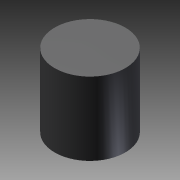
# Autodesk Inventor part: MB2011S-plunger
Saved by Autodesk Inventor 2015 (Build 190159000, 159)
## iProperties
Category: PARTsolutions
Company: NKKSWITCHES
Created: 2015-01-04
Part Number: MB2011S-plunger
Catalog Web Link: www.cadenas.de
Description: MB2000 Series - Bushing Mount Miniature Pushbuttons -plunger-
Vendor: NKKSWITCHES
Document SubType Name: Modeling
Designer: PARTuser1
Manufacturer: NKKSWITCHES
Mass: 0.0197371 g
Surface Area: 0.404353 cm^2
Volume: 0.0197371 cm^3
Density: 1 g/cm^3
Material: Generic
Appearance: PSOLRGB-192-192-192
PSOL_IDENT_0: {$CADENAS_DATA\23d-libs\nkkswitches\pushbuttons\mb2000\parts\mb2000_bm_plunger.prj},244 {VTYP=3D},{N
PSOL_IDENT_1: B=MB2011S-plunger},{LINA=MB2011S-plunger},{NN=MB2000 Series - Bushing Mount Miniature Pushbuttons -p
PSOL_IDENT_2: lunger},{DATE=21.11.2014 08:56:24},{GEOMDATE=18.02.2009 11:29:00},{VERSION=},{LINEID=10},{LINESUBID=
PSOL_IDENT_3: -1},{WBVAR=PLSCRCTS,PLNGRTYPS}  {NB=MB2011S-plunger},{LINA=MB2011S-plunger},{KT=DUMMY},{PN=MB2011S},
PSOL_IDENT_4: {SRS=MB},{PLSCRCTS=2011},{PLNGRTYPS=S},{H=0.118},{HCP=0.091}
SUPPLIER: NKKSWITCHES
ARTICLENO: MB2011S-plunger
BOMINFO: MB2011S-plunger
CREATOR: CADENAS GmbH
Title: MB2011S-plunger
Author: Cadenas PARTsolutions
Autodesk Inventor part; units mm, degrees
sketch "Sketch_1" plane through (0, 0, 0) normal (1, 0, 0) x (0, 1, 0)
  line L0 (0, 0) -> (2.9972, 0)
  line L1 (2.9972, 0) -> (2.9972, -1.4478)
  line L2 (2.9972, -1.4478) -> (0, -1.4478)
  line L3 (0, -1.4478) -> (0, 0)
  line L4 (0, 0) -> (2.9972, 0)
  constraints: 10 end point
revolve "Revolution1" add sketch "Sketch_1" angle 360 about axis through (0, 0, 0) along (0, -1, 0)
ref_plane "to_bushing_XY" through (0, 0, 0) normal (0, 1, 0) x (1, 0, 0)
ref_plane "to_bushing_YZ" through (0, 0, 0) normal (1, 0, 0) x (0, 0, -1)
ref_plane "to_bushing_ZX" through (0, 0, 0) normal (0, 0, -1) x (0, 1, 0)
ref_plane "to_caps_S_XY" through (0, 2.3114, 0) normal (0, 1, 0) x (1, 0, 0)
ref_plane "to_caps_S_YZ" through (0, 2.3114, 0) normal (1, 0, 0) x (0, 0, -1)
ref_plane "to_caps_S_ZX" through (0, 2.3114, 0) normal (0, 0, -1) x (0, 1, 0)
body "Solid1"
